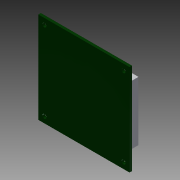
# Autodesk Inventor part: SFE-ProcessingBoard01
Saved by Autodesk Inventor 2013 (Build 170138000, 138)
## iProperties
Created: 2014-04-13
Part Number: SFE-ProcessingBoard01
Material: PCB(1)
Document SubType Name: Modeling
Designer: spichelh
Density: 1 g/cm^3
Author: spichelh
Autodesk Inventor part; units mm, degrees
ref_plane "YZ Plane" through (0, 0, 0) normal (1, 0, 0) x (0, 1, 0)
ref_plane "XZ Plane" through (0, 0, 0) normal (0, 1, 0) x (-1, 0, 0)
ref_plane "XY Plane" through (0, 0, 0) normal (0, 0, 1) x (1, 0, 0)
sketch "Sketch1" plane through (0, 0, 0) normal (0, 0, 1) x (1, 0, 0)
  line L0 (-28.575, -28.575) -> (28.575, -28.575)
  line L1 (28.575, -28.575) -> (28.575, 28.575)
  line L2 (28.575, 28.575) -> (-28.575, 28.575)
  line L3 (-28.575, 28.575) -> (-28.575, -28.575)
  line L4 (-28.575, -28.575) -> (28.575, 28.575) construction
  line L5 (28.575, -28.575) -> (-28.575, 28.575) construction
  line L6 (-28.575, 0) -> (28.575, 0) construction
  line L7 (0, 28.575) -> (0, -28.575) construction
  circle A0 centre (-24.765, 24.765) radius 1.3
  circle A1 centre (24.765, 24.765) radius 1.3
  circle A2 centre (-24.765, -24.765) radius 1.3
  circle A3 centre (24.765, -24.765) radius 1.3
  point P0 (0, 0)
  dimension "d2" = 57.15
  dimension "d4" = 57.15
  dimension "d26" = 2.6
  dimension "d27" = 3.81
  constraints: 16 end point, 6 midpoint, 4 centre point, 3 symmetric about line, 2 parallel, 1 horizontal, 1 perpendicular, 1 point on line, 3 other
  measures "d2" distance of L1.end L2.end
  measures "d4" distance of L0.end L1.end
  measures "d26" diameter of A0
  measures "d27" distance from line of L2 A0.centre
extrude "Extrusion1" add sketch "Sketch1" along normal blind 1.6
sketch "Sketch4" plane through (0, 0, 0) normal (0, 0, -1) x (-1, 0, 0)
  line L0 (-28.575, -28.575) -> (28.575, -28.575)
  line L1 (-28.575, 28.575) -> (-28.575, -28.575)
  line L2 (-26.575, 18.5) -> (-20.275, 18.5)
  line L3 (-20.275, 18.5) -> (-20.275, -18.5)
  line L4 (-20.275, -18.5) -> (-26.575, -18.5)
  line L5 (-26.575, -18.5) -> (-26.575, 18.5)
  line L6 (-20.275, 18.5) -> (-26.575, -18.5) construction
  line L7 (-26.575, 18.5) -> (-20.275, -18.5) construction
  line L8 (0, 0) -> (-28.575, 0) construction
  line L9 (0, -28.575) -> (0, 0) construction
  line L10 (26.575, 18.5) -> (20.275, 18.5)
  line L11 (20.275, 18.5) -> (20.275, -18.5)
  line L12 (20.275, -18.5) -> (26.575, -18.5)
  line L13 (26.575, -18.5) -> (26.575, 18.5)
  line L14 (28.575, -28.575) -> (-28.575, -28.575) projected
  line L15 (28.575, 28.575) -> (28.575, -28.575) projected
  line L16 (-28.575, 28.575) -> (28.575, 28.575) projected
  line L17 (-28.575, -28.575) -> (-28.575, 28.575) projected
  point P0 (-23.425, 0)
  dimension "d21" = 37
  dimension "d22" = 6.3
  dimension "d23" = 2
  constraints: 28 end point, 4 symmetric about line, 3 midpoint, 2 parallel, 2 perpendicular, 1 horizontal, 1 point on line
  measures "d21" distance of L2.end L3.end
  measures "d22" distance between parallel lines of L5 L3
  measures "d23" distance between parallel lines of L1 L5
extrude "Extrusion4" add sketch "Sketch4" along normal blind 6 contours L2 L3 L4 L5 | L13 L12 L11 L10
body "Solid1"
